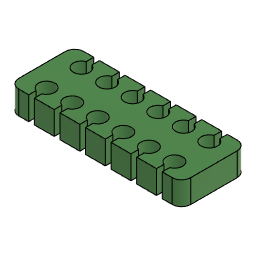
Tiny Cable Comb v5 (Autodesk Fusion 360 design; units mm, degrees)
Autodesk Fusion 360 part; units mm, degrees
sketch "Sketch1" plane through (0, 0, 0) normal (0, 0, 1) x (1, 0, 0)
  line L0 (0, 0) -> (1.574382, 0) construction
  line L1 (0, 0) -> (0, 3.5)
  line L2 (0, 3.5) -> (3.75, 3.5)
  line L3 (3.75, 3.5) -> (3.75, 0)
  circle A0 centre (1.875, 1.875) radius 0.875
  line L4 (3.75, 1.875) -> (0, 1.875) construction
  line L5 (1.875, 1.875) -> (1.875, 3.5) construction
  line L6 (1.56875, 3.5) -> (1.56875, 2.694656)
  line L7 (2.18125, 3.5) -> (2.18125, 2.694656)
  line L8 (1.875, 1.875) -> (1.875, 1) construction
  line L9 (0, 0) -> (0, -3.5)
  line L10 (0, -3.5) -> (3.75, -3.5)
  line L11 (1.56875, -3.5) -> (1.56875, -2.694656)
  line L12 (2.18125, -3.5) -> (2.18125, -2.694656)
  circle A1 centre (1.875, -1.875) radius 0.875
  line L13 (3.75, -3.5) -> (3.75, 0)
  point P0 (1, 1.875)
  point P1 (1.875, 1)
  point P2 (1.875, 2.75)
  dimension "d20" = 1.75
  dimension "d21" = 1
  dimension "d22" = 0.6125
  dimension "d24" = 0.75
  dimension "d25" = 1
  constraint coincident L0.start L1.start
  constraint horizontal L0
  constraint perpendicular L0 L1
  constraint perpendicular L1 L2
  constraint coincident L0 L3.end
  constraint perpendicular L0 L3
  constraint coincident L3 L4.start
  constraint coincident L1 L4.end
  constraint perpendicular L1 L4
  constraint midpoint A0.centre L4
  constraint coincident A0 P0
  constraint coincident L4 P0
  constraint coincident A0.centre L5.start
  constraint midpoint L2 L5.end
  constraint perpendicular L2 L6
  constraint perpendicular L2 L7
  constraint symmetric L5 L6 L7
  constraint coincident A0 P1
  constraint perpendicular L4 L8
  constraint coincident P1 L8.end
  constraint coincident A0 P2
  constraint coincident L5 P2
  constraint symmetric L1.start L0 L9.start
  constraint symmetric L0 L1.end L9.end
  constraint symmetric L0 L2.end L10.end
  constraint symmetric L0 L3.end L13.end
  constraint symmetric L0 A0 A1
  measures "d20" diameter of A0
  measures "d21" distance of L4.end P0
  measures "d22" distance of L6 L7
  measures "d24" distance of L2 P2
  measures "d25" distance of L0 P1
extrude "Extrude1" add sketch "Sketch1" along normal blind 2.5 contours L1 L2 L3 A0 L6 L7 L9 L10 L11 L12 A1 L13 picked at (1.068558, 0) makes body 1
pattern_linear "R-Pattern1" count 6 spacing 2.75 along (1, 0, 0) of "Extrude1" makes body 2 makes body 3 makes body 4 makes body 5 makes body 6
combine "Combine1" operation add target body 1 tool bodies 2 4 5 3 6
extrude "Extrude2" add 1 faces at (0, -1.166667, 0.833333) along direction (-1, 0, 0) blind 0.5 on bodies 1 bodies 1
extrude "Extrude3" add 1 faces at (17.5, 1.166667, 0.833333) along direction (1, 0, 0) blind 0.5 on bodies 1 bodies 1
fillet "Fillet1" radius 1 4 edges at (18, -3.5, 1.25) (18, 3.5, 1.25) (-0.5, 3.5, 1.25) (-0.5, -3.5, 1.25) on bodies 1
equation "wireDiameter = 1.75 mm"
equation "toothSize = 1 mm"
equation "d16 = toothSize + wireDiameter"
equation "d20 = wireDiameter"
equation "d21 = toothSize"
equation "d22 = wireDiameter * 0.35"
equation "d24 = toothSize * 0.75"
equation "d25 = toothSize"
equation "d31 = toothSize"
